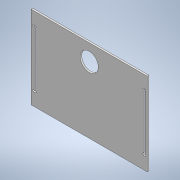
# Autodesk Inventor part: body_top
Saved by Autodesk Inventor 2022 (Build 260153000, 153)
## iProperties
Created: 2022-10-18
Part Number: body_top
Material: 一般
Document SubType Name: Modeling
Designer: haya
Density: 1 g/cm^3
Appearance: 既定
Author: haya
Autodesk Inventor part; units mm, degrees
ref_plane "YZ Plane" through (0, 0, 0) normal (1, 0, 0) x (0, 1, 0)
ref_plane "XZ Plane" through (0, 0, 0) normal (0, 1, 0) x (-1, 0, 0)
ref_plane "XY Plane" through (0, 0, 0) normal (0, 0, 1) x (1, 0, 0)
sketch "スケッチ1" plane through (0, 0, 0) normal (0, 0, 1) x (1, 0, 0)
  line L0 (0, 0) -> (140, 0)
  line L1 (140, 0) -> (140, 100)
  line L2 (140, 100) -> (0, 100)
  line L3 (0, 100) -> (0, 0)
  dimension "d0" = 140
  dimension "d1" = 100
  constraints: 8 end point, 2 parallel, 1 horizontal, 1 perpendicular
  measures "d0" distance of L0.start L0.end
  measures "d1" distance of L2.end L0.start
extrude "押し出し1" add sketch "スケッチ1" along normal blind 2
sketch "スケッチ2" plane through (0, 0, 2) normal (0, 0, 1) x (1, 0, 0)
  line L0 (140, 100) -> (0, 100) projected
  line L1 (70, 100) -> (70, 0) construction
  line L2 (0, 0) -> (140, 0) projected
  line L3 (2.5, 85) -> (5, 85)
  line L4 (5, 83) -> (5, 17)
  line L5 (5, 15) -> (2.5, 15)
  line L6 (2.5, 17) -> (2.5, 83)
  line L7 (0, 100) -> (0, 0) projected
  line L8 (0, 50) -> (140, 50) construction
  line L9 (140, 0) -> (140, 100) projected
  arc A0 (2.5, 85) -> (2.5, 83) centre (2.5, 84) ccw
  arc A1 (5, 83) -> (5, 85) centre (5, 84) ccw
  arc A2 (2.5, 17) -> (2.5, 15) centre (2.5, 16) ccw
  arc A3 (5, 15) -> (5, 17) centre (5, 16) ccw
  line L10 (137.5, 85) -> (135, 85)
  line L11 (135, 83) -> (135, 17)
  line L12 (135, 15) -> (137.5, 15)
  line L13 (137.5, 17) -> (137.5, 83)
  line L14 (140, 50) -> (0, 50) construction
  arc A4 (137.5, 83) -> (137.5, 85) centre (137.5, 84) ccw
  arc A5 (135, 85) -> (135, 83) centre (135, 84) ccw
  arc A6 (137.5, 15) -> (137.5, 17) centre (137.5, 16) ccw
  arc A7 (135, 17) -> (135, 15) centre (135, 16) ccw
  dimension "d4" = 2.5
  dimension "d5" = 2.5
  dimension "d6" = 70
  dimension "d7" = 2
  dimension "d8" = 2
  dimension "d9" = 2
  dimension "d10" = 2
  constraints: 22 end point, 16 point on circle, 14 symmetric about line, 8 centre point, 8 point on line, 4 midpoint, 2 parallel, 1 horizontal, 1 perpendicular, 5 other
  measures "d4" distance between parallel lines of L6 L7
  measures "d5" distance between parallel lines of L6 L4
  measures "d6" distance of L5.end L3.start
  measures "d7" diameter of A0
  measures "d8" diameter of A1
  measures "d9" diameter of A2
  measures "d10" diameter of A3
extrude "押し出し2" cut sketch "スケッチ2" against normal through all contours L3 A1 L4 A3 L5 A2 L6 A0 | A4 L13 A6 L12 A7 L11 A5 L10
sketch "スケッチ3" plane through (0, 0, 2) normal (0, 0, 1) x (1, 0, 0)
  line L0 (140, 100) -> (0, 100) projected
  line L1 (70, 100) -> (70, 0) construction
  line L2 (0, 0) -> (140, 0) projected
  point P0 (70, 80)
  dimension "d13" = 20
  constraints: 2 end point, 2 midpoint, 1 point on line
  measures "d13" distance from line of point (70, 80) L0
hole "穴1" at (70, 80, 2) direction (0, 0, -1) diameter 22 end through all
